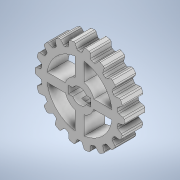
# Autodesk Inventor part: center_gear
Saved by Autodesk Inventor 2022 (Build 260153000, 153)
## iProperties
Created: 2022-06-21
Part Number: center_gear
Material: Generic
Document SubType Name: Modeling
Designer: efred
Density: 1 g/cm^3
Appearance: Default
Author: efred
Autodesk Inventor part; units mm, degrees
ref_plane "YZ Plane" through (0, 0, 0) normal (1, 0, 0) x (0, 1, 0)
ref_plane "XZ Plane" through (0, 0, 0) normal (0, 1, 0) x (-1, 0, 0)
ref_plane "XY Plane" through (0, 0, 0) normal (0, 0, 1) x (1, 0, 0)
sketch "Sketch1" plane through (0, 0, 0) normal (0, 0, 1) x (1, 0, 0)
  circle A0 centre (0, 0) radius 0.5 projected
  line L0 (-1.1547, -2) -> (-1.7321, -1) projected
  line L1 (-1.7321, -1) -> (-3.5, -1) projected
  line L2 (-3.5, -1) -> (-3.5, 1) projected
  line L3 (-3.5, 1) -> (-1.7321, 1) projected
  line L4 (-1.7321, 1) -> (-1.1547, 2) projected
  line L5 (-1.1547, 2) -> (1.1547, 2) projected
  line L6 (1.1547, 2) -> (1.7321, 1) projected
  line L7 (1.7321, 1) -> (3.5, 1) projected
  line L8 (3.5, 1) -> (3.5, -1) projected
  line L9 (3.5, -1) -> (1.7321, -1) projected
  line L10 (1.7321, -1) -> (1.1547, -2) projected
  line L11 (1.1547, -2) -> (-1.1547, -2) projected
  circle A1 centre (0, 0) radius 5
  line L12 (-3.8, -1.3) -> (-1.9053, -1.3)
  line L13 (-1.9053, -1.3) -> (-1.3279, -2.3)
  line L14 (-1.3279, -2.3) -> (1.3279, -2.3)
  line L15 (1.3279, -2.3) -> (1.9053, -1.3)
  line L16 (1.9053, -1.3) -> (3.8, -1.3)
  line L17 (3.8, -1.3) -> (3.8, 1.3)
  line L18 (3.8, 1.3) -> (1.9053, 1.3)
  line L19 (1.9053, 1.3) -> (1.3279, 2.3)
  line L20 (1.3279, 2.3) -> (-1.3279, 2.3)
  line L21 (-1.3279, 2.3) -> (-1.9053, 1.3)
  line L22 (-1.9053, 1.3) -> (-3.8, 1.3)
  line L23 (-3.8, 1.3) -> (-3.8, -1.3)
  dimension "d0" = 10
  dimension "d1" = 0.3
  constraints: 24 end point, 1 centre point, 1 coincident, 11 other
  measures "d0" diameter of A1
  measures "d1" distance between parallel lines of L1 L12
extrude "Extrusion1" add sketch "Sketch1" along normal blind 2 and the other way blind 5 contours A1
sketch "Sketch2" plane through (0, 0, -5) normal (0, 0, -1) x (-1, 0, 0)
  circle A0 centre (0, 0) radius 5 projected
  line L0 (3.8, 1.3) -> (3.8, -1.3) projected
  line L1 (3.8, -1.3) -> (1.9053, -1.3) projected
  line L2 (1.9053, -1.3) -> (1.3279, -2.3) projected
  line L3 (1.3279, -2.3) -> (-1.3279, -2.3) projected
  line L4 (-1.3279, -2.3) -> (-1.9053, -1.3) projected
  line L5 (-1.9053, -1.3) -> (-3.8, -1.3) projected
  line L6 (-3.8, -1.3) -> (-3.8, 1.3) projected
  line L7 (-3.8, 1.3) -> (-1.9053, 1.3) projected
  line L8 (-1.9053, 1.3) -> (-1.3279, 2.3) projected
  line L9 (-1.3279, 2.3) -> (1.3279, 2.3) projected
  line L10 (1.3279, 2.3) -> (1.9053, 1.3) projected
  line L11 (1.9053, 1.3) -> (3.8, 1.3) projected
  line L12 (3.8, 1.3) -> (3.8, -1.3) projected
  line L13 (3.8, 1.3) -> (3.8, -1.3)
  line L14 (3.8, -1.3) -> (1.9053, -1.3)
  line L15 (1.9053, -1.3) -> (1.3279, -2.3) projected
  line L16 (1.9053, -1.3) -> (1.3279, -2.3)
  line L17 (-1.9053, -1.3) -> (-1.3279, -2.3) projected
  line L18 (-1.3279, -2.3) -> (1.3279, -2.3)
  line L19 (1.9053, 1.3) -> (3.8, 1.3) projected
  line L20 (3.8, 1.3) -> (1.9053, 1.3)
  line L21 (1.3279, 2.3) -> (1.9053, 1.3) projected
  line L22 (1.9053, 1.3) -> (1.3279, 2.3)
  line L23 (1.3279, 2.3) -> (-1.3279, 2.3)
  line L24 (-1.3, 1.9053) -> (-2.3, 1.3279)
  line L25 (-2.3, 1.3279) -> (-2.3, -1.3279)
  line L26 (2.3, -1.3279) -> (2.3, 1.3279)
  line L27 (1.3, 1.9053) -> (2.3, 1.3279)
  line L28 (1.3, 3.8) -> (1.3, 1.9053)
  line L29 (-1.3, 3.8) -> (-1.3, 1.9053)
  line L30 (-1.3, 3.8) -> (1.3, 3.8)
  line L31 (-1.9053, -1.3) -> (-1.3279, -2.3)
  line L32 (-1.3279, -2.3) -> (1.3279, -2.3)
  line L33 (1.3279, 2.3) -> (-1.3279, 2.3)
  line L34 (-1.9053, 1.3) -> (-1.3279, 2.3)
  line L35 (-3.8, 1.3) -> (-1.9053, 1.3)
  line L36 (-3.8, -1.3) -> (-1.9053, -1.3)
  line L37 (-3.8, -1.3) -> (-3.8, 1.3)
  line L38 (1.3, -1.9053) -> (2.3, -1.3279)
  line L39 (2.3, -1.3279) -> (2.3, 1.3279)
  line L40 (-2.3, 1.3279) -> (-2.3, -1.3279)
  line L41 (-1.3, -1.9053) -> (-2.3, -1.3279)
  line L42 (-1.3, -3.8) -> (-1.3, -1.9053)
  line L43 (1.3, -3.8) -> (1.3, -1.9053)
  line L44 (1.3, -3.8) -> (-1.3, -3.8)
  point P0 (1.3, -2.3)
  point P1 (-1.3, -2.3)
  point P2 (-1.3, 2.3)
  point P3 (1.3, 2.3)
  point P4 (-2.3, 1.3)
  point P5 (-1.6837, 1.6837)
  point P6 (-1.6837, -1.6837)
  point P7 (-2.3, -1.3)
  point P8 (1.6837, -1.6837)
  point P9 (2.3, -1.3)
  point P10 (1.6837, 1.6837)
  point P11 (2.3, 1.3)
  dimension "d8" = 360
  constraints: 56 end point, 4 collinear, 1 point on line, 65 other
ref_plane "Work Plane1" through (-8.8, -2.2, 0) normal (0, 0, 1) x (1, 0, 0)
extrude "Extrusion2" cut sketch "Sketch2" against normal up to surface (5 mm away) contours L11 L10 L27 L26 | L26 L38 L2 L1 | L9 L29 L30 L28 | L43 L44 L42 L3 | L8 L7 L25 L24 | L41 L25 L5 L4
sketch "Sketch3" plane through (0, 0, -5) normal (0, 0, -1) x (-1, 0, 0)
  line L0 (-1.6837, 1.6837) -> (-2.3, 1.3279) projected
  circle A0 centre (0, 0) radius 2.6558
  constraints: 1 coincident, 3 other
extrude "Extrusion3" cut sketch "Sketch3" against normal through all
sketch "Sketch4" plane through (0, 0, -5) normal (0, 0, -1) x (-1, 0, 0)
  circle A0 centre (0, 0) radius 5 projected
  circle A1 centre (0, 0) radius 15 construction
  circle A2 centre (-20.3143, -27.9603) radius 16.5 construction
  circle A3 centre (0, 0) radius 13
  circle A4 centre (0, 0) radius 11
  line L0 (-12.9132, -1.5) -> (-4.7697, -1.5)
  line L1 (-4.7697, -1.5) -> (-4.7697, 1.5)
  line L2 (-4.7697, 1.5) -> (-12.9132, 1.5)
  line L3 (-12.9132, 1.5) -> (-12.9132, -1.5)
  line L4 (-5, 0) -> (-11, 0) construction
  line L5 (1.5, -12.9132) -> (1.5, -4.7697)
  line L6 (-1.5, -4.7697) -> (-1.5, -12.9132)
  line L7 (12.9132, 1.5) -> (4.7697, 1.5)
  line L8 (4.7697, -1.5) -> (12.9132, -1.5)
  line L9 (-1.5, 12.9132) -> (-1.5, 4.7697)
  line L10 (1.5, 4.7697) -> (1.5, 12.9132)
  line L11 (-14.6058, -1.0879) -> (-12.9132, -1.5)
  line L12 (-14.6058, 1.0879) -> (-12.9132, 1.5)
  arc A5 (-14.9871, 0.6228) -> (-14.9871, -0.6228) centre (0, 0) ccw
  arc A6 (-14.9871, -0.6228) -> (-14.6058, -1.0879) centre (-14.4875, -0.6021) ccw
  arc A7 (-14.6058, 1.0879) -> (-14.9871, 0.6228) centre (-14.4875, 0.6021) ccw
  arc A8 (-13.2467, 1.4188) -> (-12.87, 1.8341) centre (-13.365, 1.9046) ccw
  arc A9 (-12.87, -1.8341) -> (-13.2467, -1.4188) centre (-13.365, -1.9046) ccw
  arc A10 (-12.9331, -3.1974) -> (-12.7211, -2.6783) centre (-13.2104, -2.7814) ccw
  line L13 (-14.097, -3.9732) -> (-12.6474, -3.007)
  arc A11 (-14.097, -3.9732) -> (-14.2962, -4.5406) centre (-13.8197, -4.3893) ccw
  arc A12 (-14.2962, -4.5406) -> (-13.8702, -5.7111) centre (0, 0) ccw
  arc A13 (-13.8702, -5.7111) -> (-13.3529, -6.0177) centre (-13.4079, -5.5208) ccw
  arc A14 (-11.4665, -6.1252) -> (-11.9626, -5.8639) centre (-11.9076, -6.3608) ccw
  line L14 (-13.3529, -6.0177) -> (-11.6214, -5.8261)
  arc A15 (-11.0595, -7.4279) -> (-11.0379, -6.8677) centre (-11.4624, -7.1318) ccw
  line L15 (-11.8879, -8.5551) -> (-10.8562, -7.1514)
  arc A16 (-11.8879, -8.5551) -> (-11.8811, -9.1564) centre (-11.4851, -8.8512) ccw
  arc A17 (-11.8811, -9.1564) -> (-11.0804, -10.1106) centre (0, 0) ccw
  arc A18 (-11.0804, -10.1106) -> (-10.4894, -10.2218) centre (-10.7111, -9.7736) ccw
  arc A19 (-8.6801, -9.6776) -> (-9.2356, -9.6017) centre (-9.0139, -10.0498) ccw
  line L16 (-10.4894, -10.2218) -> (-8.9279, -9.4495)
  arc A20 (-7.8521, -10.7626) -> (-8.0233, -10.2287) centre (-8.3319, -10.6221) ccw
  line L17 (-8.245, -12.105) -> (-7.7556, -10.4331)
  arc A21 (-8.245, -12.105) -> (-8.0329, -12.6678) centre (-7.7651, -12.2455) ccw
  arc A22 (-8.0329, -12.6678) -> (-6.9542, -13.2906) centre (0, 0) ccw
  arc A23 (-6.9542, -13.2906) -> (-6.3608, -13.1929) centre (-6.7224, -12.8476) ccw
  arc A24 (-4.8466, -12.0628) -> (-5.3946, -12.1814) centre (-5.0331, -12.5267) ccw
  line L18 (-6.3608, -13.1929) -> (-5.1575, -11.9331)
  arc A25 (-3.6975, -12.7991) -> (-4.041, -12.356) centre (-4.1965, -12.8312) ccw
  line L19 (-3.6076, -14.195) -> (-3.7196, -12.4565)
  arc A26 (-3.6076, -14.195) -> (-3.2158, -14.6512) centre (-3.1086, -14.1629) ccw
  arc A27 (-3.2158, -14.6512) -> (-1.9891, -14.8675) centre (0, 0) ccw
  arc A28 (-1.9891, -14.8675) -> (-1.4649, -14.5728) centre (-1.9228, -14.3719) ccw
  arc A29 (-0.4287, -12.9929) -> (-0.903, -13.2918) centre (-0.4451, -13.4927) ccw
  line L20 (-1.4649, -14.5728) -> (-0.7651, -12.9775)
  arc A30 (0.903, -13.2918) -> (0.4287, -12.9929) centre (0.4451, -13.4927) ccw
  line L21 (1.4649, -14.5728) -> (0.7651, -12.9775)
  arc A31 (1.4649, -14.5728) -> (1.9891, -14.8675) centre (1.9228, -14.3719) ccw
  arc A32 (1.9891, -14.8675) -> (3.2158, -14.6512) centre (0, 0) ccw
  arc A33 (3.2158, -14.6512) -> (3.6076, -14.195) centre (3.1086, -14.1629) ccw
  arc A34 (4.041, -12.356) -> (3.6975, -12.7991) centre (4.1965, -12.8312) ccw
  line L22 (3.6076, -14.195) -> (3.7196, -12.4565)
  arc A35 (5.3946, -12.1814) -> (4.8466, -12.0628) centre (5.0331, -12.5267) ccw
  line L23 (6.3608, -13.1929) -> (5.1575, -11.9331)
  arc A36 (6.3608, -13.1929) -> (6.9542, -13.2906) centre (6.7224, -12.8476) ccw
  arc A37 (6.9542, -13.2906) -> (8.0329, -12.6678) centre (0, 0) ccw
  arc A38 (8.0329, -12.6678) -> (8.245, -12.105) centre (7.7651, -12.2455) ccw
  arc A39 (8.0233, -10.2287) -> (7.8521, -10.7626) centre (8.3319, -10.6221) ccw
  line L24 (8.245, -12.105) -> (7.7556, -10.4331)
  arc A40 (9.2356, -9.6017) -> (8.6801, -9.6776) centre (9.0139, -10.0498) ccw
  line L25 (10.4894, -10.2218) -> (8.9279, -9.4495)
  arc A41 (10.4894, -10.2218) -> (11.0804, -10.1106) centre (10.7111, -9.7736) ccw
  arc A42 (11.0804, -10.1106) -> (11.8811, -9.1564) centre (0, 0) ccw
  arc A43 (11.8811, -9.1564) -> (11.8879, -8.5551) centre (11.4851, -8.8512) ccw
  arc A44 (11.0379, -6.8677) -> (11.0595, -7.4279) centre (11.4624, -7.1318) ccw
  line L26 (11.8879, -8.5551) -> (10.8562, -7.1514)
  arc A45 (11.9626, -5.8639) -> (11.4665, -6.1252) centre (11.9076, -6.3608) ccw
  line L27 (13.3529, -6.0177) -> (11.6214, -5.8261)
  arc A46 (13.3529, -6.0177) -> (13.8702, -5.7111) centre (13.4079, -5.5208) ccw
  arc A47 (13.8702, -5.7111) -> (14.2962, -4.5406) centre (0, 0) ccw
  arc A48 (14.2962, -4.5406) -> (14.097, -3.9732) centre (13.8197, -4.3893) ccw
  arc A49 (12.7211, -2.6783) -> (12.9331, -3.1974) centre (13.2104, -2.7814) ccw
  line L28 (14.097, -3.9732) -> (12.6474, -3.007)
  arc A50 (13.2467, -1.4188) -> (12.87, -1.8341) centre (13.365, -1.9046) ccw
  line L29 (14.6058, -1.0879) -> (12.9132, -1.5)
  arc A51 (14.6058, -1.0879) -> (14.9871, -0.6228) centre (14.4875, -0.6021) ccw
  arc A52 (14.9871, -0.6228) -> (14.9871, 0.6228) centre (0, 0) ccw
  arc A53 (14.9871, 0.6228) -> (14.6058, 1.0879) centre (14.4875, 0.6021) ccw
  arc A54 (12.87, 1.8341) -> (13.2467, 1.4188) centre (13.365, 1.9046) ccw
  line L30 (14.6058, 1.0879) -> (12.9132, 1.5)
  arc A55 (12.9331, 3.1974) -> (12.7211, 2.6783) centre (13.2104, 2.7814) ccw
  line L31 (14.097, 3.9732) -> (12.6474, 3.007)
  arc A56 (14.097, 3.9732) -> (14.2962, 4.5406) centre (13.8197, 4.3893) ccw
  arc A57 (14.2962, 4.5406) -> (13.8702, 5.7111) centre (0, 0) ccw
  arc A58 (13.8702, 5.7111) -> (13.3529, 6.0177) centre (13.4079, 5.5208) ccw
  arc A59 (11.4665, 6.1252) -> (11.9626, 5.8639) centre (11.9076, 6.3608) ccw
  line L32 (13.3529, 6.0177) -> (11.6214, 5.8261)
  arc A60 (11.0595, 7.4279) -> (11.0379, 6.8677) centre (11.4624, 7.1318) ccw
  line L33 (11.8879, 8.5551) -> (10.8562, 7.1514)
  arc A61 (11.8879, 8.5551) -> (11.8811, 9.1564) centre (11.4851, 8.8512) ccw
  arc A62 (11.8811, 9.1564) -> (11.0804, 10.1106) centre (0, 0) ccw
  arc A63 (11.0804, 10.1106) -> (10.4894, 10.2218) centre (10.7111, 9.7736) ccw
  arc A64 (8.6801, 9.6776) -> (9.2356, 9.6017) centre (9.0139, 10.0498) ccw
  line L34 (10.4894, 10.2218) -> (8.9279, 9.4495)
  arc A65 (7.8521, 10.7626) -> (8.0233, 10.2287) centre (8.3319, 10.6221) ccw
  line L35 (8.245, 12.105) -> (7.7556, 10.4331)
  arc A66 (8.245, 12.105) -> (8.0329, 12.6678) centre (7.7651, 12.2455) ccw
  arc A67 (8.0329, 12.6678) -> (6.9542, 13.2906) centre (0, 0) ccw
  arc A68 (6.9542, 13.2906) -> (6.3608, 13.1929) centre (6.7224, 12.8476) ccw
  arc A69 (4.8466, 12.0628) -> (5.3946, 12.1814) centre (5.0331, 12.5267) ccw
  line L36 (6.3608, 13.1929) -> (5.1575, 11.9331)
  arc A70 (3.6975, 12.7991) -> (4.041, 12.356) centre (4.1965, 12.8312) ccw
  line L37 (3.6076, 14.195) -> (3.7196, 12.4565)
  arc A71 (3.6076, 14.195) -> (3.2158, 14.6512) centre (3.1086, 14.1629) ccw
  arc A72 (3.2158, 14.6512) -> (1.9891, 14.8675) centre (0, 0) ccw
  arc A73 (1.9891, 14.8675) -> (1.4649, 14.5728) centre (1.9228, 14.3719) ccw
  arc A74 (0.4287, 12.9929) -> (0.903, 13.2918) centre (0.4451, 13.4927) ccw
  line L38 (1.4649, 14.5728) -> (0.7651, 12.9775)
  arc A75 (-0.903, 13.2918) -> (-0.4287, 12.9929) centre (-0.4451, 13.4927) ccw
  line L39 (-1.4649, 14.5728) -> (-0.7651, 12.9775)
  arc A76 (-1.4649, 14.5728) -> (-1.9891, 14.8675) centre (-1.9228, 14.3719) ccw
  arc A77 (-1.9891, 14.8675) -> (-3.2158, 14.6512) centre (0, 0) ccw
  arc A78 (-3.2158, 14.6512) -> (-3.6076, 14.195) centre (-3.1086, 14.1629) ccw
  arc A79 (-4.041, 12.356) -> (-3.6975, 12.7991) centre (-4.1965, 12.8312) ccw
  line L40 (-3.6076, 14.195) -> (-3.7196, 12.4565)
  arc A80 (-5.3946, 12.1814) -> (-4.8466, 12.0628) centre (-5.0331, 12.5267) ccw
  line L41 (-6.3608, 13.1929) -> (-5.1575, 11.9331)
  arc A81 (-6.3608, 13.1929) -> (-6.9542, 13.2906) centre (-6.7224, 12.8476) ccw
  arc A82 (-6.9542, 13.2906) -> (-8.0329, 12.6678) centre (0, 0) ccw
  arc A83 (-8.0329, 12.6678) -> (-8.245, 12.105) centre (-7.7651, 12.2455) ccw
  arc A84 (-8.0233, 10.2287) -> (-7.8521, 10.7626) centre (-8.3319, 10.6221) ccw
  line L42 (-8.245, 12.105) -> (-7.7556, 10.4331)
  arc A85 (-9.2356, 9.6017) -> (-8.6801, 9.6776) centre (-9.0139, 10.0498) ccw
  line L43 (-10.4894, 10.2218) -> (-8.9279, 9.4495)
  arc A86 (-10.4894, 10.2218) -> (-11.0804, 10.1106) centre (-10.7111, 9.7736) ccw
  arc A87 (-11.0804, 10.1106) -> (-11.8811, 9.1564) centre (0, 0) ccw
  arc A88 (-11.8811, 9.1564) -> (-11.8879, 8.5551) centre (-11.4851, 8.8512) ccw
  arc A89 (-11.0379, 6.8677) -> (-11.0595, 7.4279) centre (-11.4624, 7.1318) ccw
  line L44 (-11.8879, 8.5551) -> (-10.8562, 7.1514)
  arc A90 (-11.9626, 5.8639) -> (-11.4665, 6.1252) centre (-11.9076, 6.3608) ccw
  line L45 (-13.3529, 6.0177) -> (-11.6214, 5.8261)
  arc A91 (-13.3529, 6.0177) -> (-13.8702, 5.7111) centre (-13.4079, 5.5208) ccw
  arc A92 (-13.8702, 5.7111) -> (-14.2962, 4.5406) centre (0, 0) ccw
  arc A93 (-14.2962, 4.5406) -> (-14.097, 3.9732) centre (-13.8197, 4.3893) ccw
  arc A94 (-12.7211, 2.6783) -> (-12.9331, 3.1974) centre (-13.2104, 2.7814) ccw
  line L46 (-14.097, 3.9732) -> (-12.6474, 3.007)
  arc A95 (-24.387, -30.8608) -> (-20.267, -32.96) centre (-20.3143, -27.9603) ccw projected
  point P0 (-14.9666, -1)
  point P1 (-14.9666, 1)
  point P2 (-14.9724, 0.9091)
  point P3 (-12.9132, 1.5)
  point P4 (-12.9132, 1.5)
  point P5 (-12.6474, -3.007)
  point P6 (-11.6214, -5.8261)
  point P7 (-8.9279, -9.4495)
  point P8 (-7.7556, -10.4331)
  point P9 (-5.1575, -11.9331)
  point P10 (-3.7196, -12.4565)
  point P11 (-0.7651, -12.9775)
  point P12 (0.7651, -12.9775)
  point P13 (3.7196, -12.4565)
  point P14 (5.1575, -11.9331)
  point P15 (7.7556, -10.4331)
  point P16 (10.8562, -7.1514)
  point P17 (11.6214, -5.8261)
  point P18 (12.6474, -3.007)
  point P19 (12.9132, -1.5)
  point P20 (12.9132, 1.5)
  point P21 (12.6474, 3.007)
  point P22 (11.6214, 5.8261)
  point P23 (10.8562, 7.1514)
  point P24 (8.9279, 9.4495)
  point P25 (7.7556, 10.4331)
  point P26 (3.7196, 12.4565)
  point P27 (0.7651, 12.9775)
  point P28 (-0.7651, 12.9775)
  point P29 (-3.7196, 12.4565)
  point P30 (-5.1575, 11.9331)
  point P31 (-8.9279, 9.4495)
  point P32 (-10.8562, 7.1514)
  point P33 (-11.6214, 5.8261)
  point P34 (-10.8972, 1.5)
  point P35 (-1.5, 10.8972)
  point P36 (-1.5, 4.7697)
  point P37 (1.5, 10.8972)
  point P38 (10.8972, 1.5)
  point P39 (4.7697, 1.5)
  point P40 (10.8972, -1.5)
  point P41 (1.5, -10.8972)
  point P42 (1.5, -4.7697)
  point P43 (-1.5, -10.8972)
  point P44 (-10.8972, -1.5)
  point P45 (-12.7211, -2.6783)
  point P46 (-11.9626, -5.8639)
  point P47 (-11.4665, -6.1252)
  point P48 (-11.0379, -6.8677)
  point P49 (-9.2356, -9.6017)
  point P50 (-8.6801, -9.6776)
  point P51 (-8.0233, -10.2287)
  point P52 (-5.3946, -12.1814)
  point P53 (-4.8466, -12.0628)
  point P54 (-4.041, -12.356)
  point P55 (-0.903, -13.2918)
  point P56 (-0.4287, -12.9929)
  point P57 (0.4287, -12.9929)
  point P58 (3.6975, -12.7991)
  point P59 (4.041, -12.356)
  point P60 (4.8466, -12.0628)
  point P61 (8.6801, -9.6776)
  point P62 (7.8521, -10.7626)
  point P63 (8.0233, -10.2287)
  point P64 (11.0595, -7.4279)
  point P65 (11.0379, -6.8677)
  point P66 (11.4665, -6.1252)
  point P67 (12.87, -1.8341)
  point P68 (12.9331, -3.1974)
  point P69 (12.7211, -2.6783)
  point P70 (13.2467, 1.4188)
  point P71 (12.87, 1.8341)
  point P72 (12.7211, 2.6783)
  point P73 (11.9626, 5.8639)
  point P74 (11.4665, 6.1252)
  point P75 (11.0379, 6.8677)
  point P76 (9.2356, 9.6017)
  point P77 (8.6801, 9.6776)
  point P78 (8.0233, 10.2287)
  point P79 (5.3946, 12.1814)
  point P80 (4.8466, 12.0628)
  point P81 (4.041, 12.356)
  point P82 (0.903, 13.2918)
  point P83 (0.4287, 12.9929)
  point P84 (-0.4287, 12.9929)
  point P85 (-3.6975, 12.7991)
  point P86 (-4.041, 12.356)
  point P87 (-4.8466, 12.0628)
  point P88 (-7.8521, 10.7626)
  point P89 (-8.0233, 10.2287)
  point P90 (-8.6801, 9.6776)
  point P91 (-11.0595, 7.4279)
  point P92 (-11.0379, 6.8677)
  point P93 (-11.4665, 6.1252)
  point P94 (-12.9331, 3.1974)
  point P95 (-12.7211, 2.6783)
  point P96 (-13.2467, -1.4188)
  point P97 (-12.87, -1.8341)
  dimension "d17" = 2
  dimension "d14" = 33
  dimension "d15" = 30
  dimension "d16" = 2
  dimension "d18" = 3
  dimension "d21" = 360
  dimension "d23" = 2
  dimension "d24" = 3
  dimension "d25" = 0.5
  dimension "d26" = 0.5
  dimension "d29" = 360
  constraints: 187 point on circle, 94 end point, 92 centre point, 20 point on line, 5 symmetric about line, 5 tangent, 2 coincident, 2 equal radius, 2 horizontal, 2 parallel, 1 horizontal alignment, 1 perpendicular, 431 other
  measures "d14" diameter of A2
  measures "d15" diameter of A1
  measures "d18" distance between parallel lines of L0 L2
  measures "d23" distance of point (-14.967, 1) A1.start
  measures "d24" distance of L11.end L12.end
  measures "d25" radius of A6
  measures "d26" radius of A8
extrude "Extrusion4" add sketch "Sketch4" against normal up to surface (7 mm away) contours A0 L7 A4 L8 | A0 L9 A4 L10 | L7 A3 L8 A4 | A4 L10 A3 L7 | L5 A4 L6 A0 | L8 A3 L5 A4 | A4 L9 A3 L10 | L30 A53 A52 A51 L29 A3 | A3 A54 L30 | L5 A3 L6 A4 | L29 A50 A3 | A0 L0 A4 L2 | A4 L2 A3 L9 | A3 L38 A73 A72 A71 L37 | L6 A3 L0 A4 | A3 L22 A33 A32 A31 L21 | A4 L0 L3 L2 | A3 L40 A78 A77 A76 L39 | L37 A70 A3 | A3 A74 L38 | A3 L31 A55 | A3 L20 A28 A27 A26 L19 | L21 A30 A3 | A3 A34 L22 | A49 L28 A3 | L12 A8 A3 | L3 A3 | A3 L11 A6 A5 A7 L12 | L39 A75 A3 | A3 A79 L40 | A3 L32 A58 A57 A56 L31 | A3 A9 L11 | L19 A25 A3 | A3 A29 L20 | L28 A48 A47 A46 L27 A3 | A69 L36 A3 | A3 A59 L32 | A3 L23 A35 | L27 A45 A3 | A94 L46 A3 | A3 L41 A80 | L36 A68 A67 A66 L35 A3 | A3 L13 A10 | A24 L18 A3 | A3 L24 A38 A37 A36 L23 | L46 A93 A92 A91 L45 A3 | A3 L42 A83 A82 A81 L41 | L35 A65 A3 | A3 L33 A60 | A3 L14 A13 A12 A11 L13 | L18 A23 A22 A21 L17 A3 | A3 A39 L24 | A44 L26 A3 | L45 A90 A3 | A3 A84 L42 | A3 L34 A63 A62 A61 L33 | A3 A14 L14 | L17 A20 A3 | L26 A43 A42 A41 L25 A3 | A64 L34 A3 | A3 L25 A40 | A89 L44 A3 | A3 L43 A85 | A3 L15 A15 | A19 L16 A3 | L44 A88 A87 A86 L43 A3 | A3 L16 A18 A17 A16 L15
body "Solid1"
